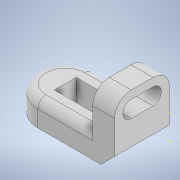
# Autodesk Inventor part: 01_01
Saved by Autodesk Inventor 2021 (Build 250183000, 183)
## iProperties
Created: 2025-03-19
Part Number: 01_01
Material: 일반
Document SubType Name: Modeling
Designer: USER
Density: 1 g/cm^3
Appearance: 기본값
Author: USER
Autodesk Inventor part; units mm, degrees
ref_plane "YZ Plane" through (0, 0, 0) normal (1, 0, 0) x (0, 1, 0)
ref_plane "XZ Plane" through (0, 0, 0) normal (0, 1, 0) x (-1, 0, 0)
ref_plane "XY Plane" through (0, 0, 0) normal (0, 0, 1) x (1, 0, 0)
sketch "스케치1" plane through (0, 0, 0) normal (0, 0, 1) x (1, 0, 0)
  point P0 (0, 0)
sketch "스케치2" plane through (0, 0, 0) normal (0, 0, 1) x (1, 0, 0)
  point P0 (0, 0)
sketch "스케치3" plane through (0, 0, 0) normal (0, 0, 1) x (1, 0, 0)
  point P0 (0, 0)
sketch "스케치4" plane through (0, 0, 0) normal (0, 0, 1) x (1, 0, 0)
  line L0 (0, 0) -> (-38, 0)
  line L1 (-38, 0) -> (-38, 9)
  line L2 (-38, 9) -> (-8, 9)
  line L3 (-8, 9) -> (-8, 23)
  line L4 (-8, 23) -> (0, 23)
  line L5 (0, 23) -> (0, 0)
  dimension "d2" = 38
  dimension "d3" = 9
  dimension "d6" = 8
  dimension "d7" = 23
  constraints: 12 end point, 4 perpendicular, 1 horizontal, 1 vertical
  measures "d2" distance of L0.start L0.end
  measures "d3" distance of L0.end L1.end
  measures "d6" distance of L3.end L4.end
  measures "d7" distance of L4.end L0.start
sketch "스케치5" plane through (0, 0, 0) normal (0, 0, 1) x (1, 0, 0)
  point P0 (0, 0)
extrude "돌출1" add sketch "스케치4" along normal blind 20
sketch "스케치6" plane through (-38, 9, 0) normal (0, 1, 0) x (1, 0, 0)
  point P0 (38, 0)
sketch "스케치7" plane through (-38, 9, 0) normal (0, 1, 0) x (1, 0, 0)
  line L0 (30, 0) -> (30, -20) projected
  line L1 (30, -14) -> (10, -14)
  line L2 (10, -14) -> (10, -6)
  line L3 (10, -6) -> (30, -6)
  line L4 (30, -6) -> (30, -14)
  line L5 (30, -20) -> (0, -20) projected
  line L6 (30, -6) -> (30, -14)
  line L7 (30, -6) -> (30, -14)
  line L8 (30, -14) -> (30, -6)
  line L9 (30, -14) -> (30, -6)
  point P0 (38, 0)
  dimension "d10" = 20
  dimension "d11" = 8
  dimension "d12" = 6
  constraints: 16 end point, 4 collinear, 2 parallel, 1 horizontal, 1 perpendicular, 1 point on line
  measures "d10" distance of L2.end L3.end
  measures "d11" distance of L1.end L2.end
  measures "d12" distance between parallel lines of L1 L5
extrude "돌출2" cut sketch "스케치7" against normal blind 10
fillet "모깎기1" radius 10 2 edges at (-38, 4.5, 20) (-38, 4.5, 0)
fillet "모깎기2" radius 6 2 edges at (-4, 23, 20) (-4, 23, 0)
sketch "스케치8" plane through (-8, 0, 6) normal (-1, 0, 0) x (0, 0, 1)
  point P0 (-6, 0)
sketch "스케치9" plane through (-8, 0, 6) normal (-1, 0, 0) x (0, 0, 1)
  point P0 (-6, 0)
sketch "스케치10" plane through (-8, 0, 6) normal (-1, 0, 0) x (0, 0, 1)
  line L0 (0, 9) -> (0, 0) projected
  line L1 (8, 9) -> (8, 0) projected
  line L2 (0, 9) -> (8, 9)
  line L3 (-6, 9) -> (14, 9) projected
  line L4 (8, 9) -> (14, 9)
  line L5 (0, 9) -> (0, 0) projected
  point P0 (-6, 0)
  constraints: 4 end point, 1 collinear, 1 horizontal, 1 perpendicular
sketch "스케치11" plane through (-8, 0, 6) normal (-1, 0, 0) x (0, 0, 1)
  line L0 (8, 9) -> (0, 9) projected
  line L1 (-6, 9) -> (0, 9) projected
  line L2 (0, 9) -> (-6, 9)
  point P0 (-6, 0)
  constraints: 2 end point, 1 collinear
sketch "스케치12" plane through (-8, 0, 6) normal (-1, 0, 0) x (0, 0, 1)
  line L0 (0, 17) -> (8, 17) construction
  line L1 (0, 14) -> (8, 14)
  line L2 (8, 20) -> (0, 20)
  arc A0 (0, 20) -> (0, 14) centre (0, 17) ccw
  arc A1 (8, 14) -> (8, 20) centre (8, 17) ccw
  line L3 (-6, 17) -> (-6, 9) projected
  line L4 (14, 0) -> (-6, 0) projected
  point P0 (4, 17)
  dimension "d18" = 8
  dimension "d19" = 6
  dimension "d20" = 10
  dimension "d21" = 17
  constraints: 8 end point, 4 point on circle, 4 tangent, 2 centre point, 1 horizontal, 1 midpoint, 1 parallel, 1 perpendicular
  measures "d18" distance of L0.start L0.end
  measures "d19" diameter of A1
  measures "d20" distance from line of point (4, 17) L3
  measures "d21" distance from line of L4 point (4, 17)
sketch "스케치13" plane through (-8, 0, 6) normal (-1, 0, 0) x (0, 0, 1)
  point P0 (-6, 0)
extrude "돌출3" cut sketch "스케치12" against normal blind 10
fillet "모깎기3" radius 3 3 edges at (-35.0711, 9, 17.0711) (-18.0001, 9, 20) (-18.0001, 9, 0)
chamfer "모따기1" distance 5 angle 45 1 edges at (0, 0, 10)
